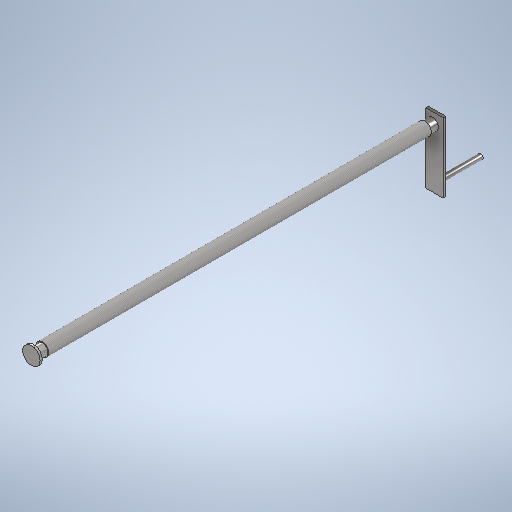
# Autodesk Inventor part: leadscrew_modified_long
Saved by Autodesk Inventor 2025.2 (Build 292293000, 293)
## iProperties
Created: 2025-01-27
Part Number: leadscrew_modified_long
Material: Steel, Alloy
Document SubType Name: Modeling
Designer: ckond
Density: 7.73 g/cm^3
Appearance: Semi-Polished
Author: ckond
Autodesk Inventor part; units mm, degrees
ref_plane "YZ Plane" through (0, 0, 0) normal (1, 0, 0) x (0, 1, 0)
ref_plane "XZ Plane" through (0, 0, 0) normal (0, 1, 0) x (-1, 0, 0)
ref_plane "XY Plane" through (0, 0, 0) normal (0, 0, 1) x (1, 0, 0)
sketch "Sketch1" plane through (0, 0, 0) normal (0, 0, 1) x (1, 0, 0)
  circle A0 centre (0, 0) radius 25
  dimension "d0" = 50
  constraints: 1 centre point, 1 coincident
  measures "d0" diameter of A0
extrude "Extrusion1" add sketch "Sketch1" along normal blind 10
sketch "Sketch2" plane through (0, 0, 10) normal (0, 0, 1) x (1, 0, 0)
  circle A0 centre (0, 0) radius 6.5
  dimension "d3" = 13
  constraints: 1 centre point, 1 coincident
  measures "d3" diameter of A0
extrude "Extrusion2" add sketch "Sketch2" along normal blind 10
fillet "Fillet1" radius 1 1 edges at (-6.5, 0, 10)
sketch "Sketch4" plane through (0, 0, 0) normal (0, 0, -1) x (-1, 0, 0)
  arc A0 (19.3649, 5) -> (5, 19.3649) centre (0, 0) ccw
  line L0 (2.5, 17.4284) -> (2.5, 9.4868)
  line L1 (9.4868, 2.5) -> (17.4284, 2.5)
  arc A1 (5, 19.3649) -> (2.5, 17.4284) centre (4.5, 17.4284) ccw
  arc A2 (17.4284, 2.5) -> (19.3649, 5) centre (17.4284, 4.5) ccw
  arc A3 (2.5, 8.3666) -> (2.5153, 8.1193) centre (4.5, 8.3666) ccw
  arc A4 (8.1193, 2.5153) -> (8.3666, 2.5) centre (8.3666, 4.5) ccw
  arc A5 (7.6798, 3.6429) -> (3.6429, 7.6798) centre (0, 0) ccw
  arc A6 (2.5, 9.4868) -> (3.6429, 7.6798) centre (4.5, 9.4868) ccw
  arc A7 (7.6798, 3.6429) -> (9.4868, 2.5) centre (9.4868, 4.5) ccw
  point P0 (2.5, 19.8431)
  point P1 (19.8431, 2.5)
  point P2 (2.5, 7.0711)
  point P3 (7.0711, 2.5)
  constraints: 20 point on circle, 10 tangent, 8 centre point, 6 point on line, 4 end point, 3 equal radius, 1 coincident
extrude "Extrusion3" cut sketch "Sketch4" against normal blind 10
pattern_circular "Circular Pattern1" count 4 over 360 about axis through (0, 0, 11) along (0, 0, -1) of "Extrusion3"
sketch "Sketch7" plane through (0, 0, 20) normal (0, 0, 1) x (1, 0, 0)
  circle A0 centre (0, 0) radius 7.5
  dimension "d38" = 15
  constraints: 1 centre point, 1 coincident
  measures "d38" diameter of A0
extrude "Extrusion5" add sketch "Sketch7" along normal blind 440
sketch "Sketch8" plane through (0, 0, 460) normal (0, 0, 1) x (1, 0, 0)
  circle A0 centre (0, 0) radius 6.5
  dimension "d41" = 13
  constraints: 1 centre point, 1 coincident
  measures "d41" diameter of A0
extrude "Extrusion6" add sketch "Sketch8" along normal blind 10
sketch "Sketch9" plane through (0, 0, 470) normal (0, 0, 1) x (1, 0, 0)
  circle A0 centre (0, 0) radius 10
  dimension "d44" = 20
  constraints: 1 centre point, 1 coincident
  measures "d44" diameter of A0
extrude "Extrusion7" add sketch "Sketch9" along normal blind 2.5
thread "Thread1" size "M15x1.5" class "6g" standard "ANSI Metric M Profile" length 440
sketch "Sketch10" plane through (0, 0, 0) normal (0, 0, -1) x (-1, 0, 0)
  circle A0 centre (0, 0) radius 25
  constraints: 1 centre point, 1 coincident
extrude "Extrusion8" cut sketch "Sketch10" against normal blind 10
sketch "Sketch11" plane through (0, 0, 10) normal (0, 0, -1) x (-1, 0, 0)
  circle A0 centre (0, 0) radius 10
  constraints: 1 centre point, 1 coincident
extrude "Extrusion9" cut sketch "Sketch11" against normal blind 1
sketch "Sketch12" plane through (0, 0, 11) normal (0, 0, -1) x (-1, 0, 0)
  circle A0 centre (0, 0) radius 3
  dimension "d53" = 6
  constraints: 1 centre point, 1 coincident
  measures "d53" diameter of A0
extrude "Extrusion10" add sketch "Sketch12" along normal blind 5
sketch "Sketch13" plane through (0, 0, 6) normal (0, 0, -1) x (-1, 0, 0)
  circle A0 centre (0, 0) radius 3 projected
  circle A1 centre (0, 0) radius 3
  line L0 (-10, 10) -> (10, 10)
  line L1 (10, 10) -> (10, -70)
  line L2 (10, -70) -> (-10, -70)
  line L3 (-10, -70) -> (-10, 10)
  dimension "d56" = 80
  constraints: 8 end point, 2 parallel, 1 centre point, 1 coincident, 1 horizontal, 1 perpendicular
  measures "d56" distance of L0.end L1.end
extrude "Extrusion11" add sketch "Sketch13" against normal blind 3
sketch "Sketch14" plane through (0, 0, 6) normal (0, 0, -1) x (-1, 0, 0)
  line L0 (10, -70) -> (-10, -70) projected
  circle A0 centre (0, -60) radius 3
  point P0 (0, 0)
  dimension "d60" = 6
  constraints: 1 centre point
  measures "d60" diameter of A0
extrude "Extrusion12" add sketch "Sketch14" along normal blind 50
body "Solid1"
